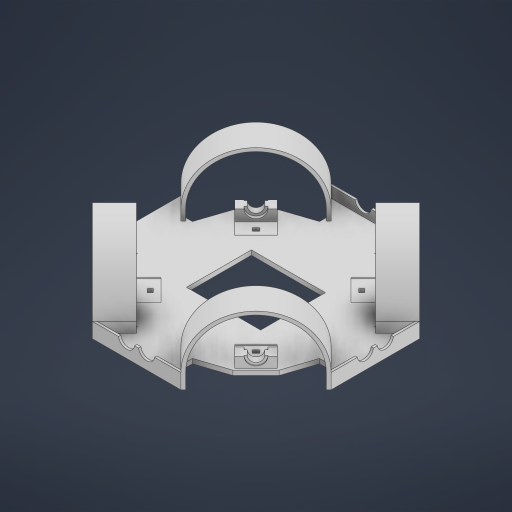
# Autodesk Inventor part: Robot Shell
Saved by Autodesk Inventor 2024 (Build 280153000, 153)
## iProperties
Created: 2025-11-14
Part Number: Robot Shell
Material: Generic
Document SubType Name: Modeling
Designer: Vincent Larson
Density: 1 g/cm^3
Appearance: Default
Author: Vincent Larson
Autodesk Inventor part; units mm, degrees
(part 1 of 2)
ref_plane "YZ Plane" through (0, 0, 0) normal (1, 0, 0) x (0, 1, 0)
ref_plane "XZ Plane" through (0, 0, 0) normal (0, 1, 0) x (-1, 0, 0)
ref_plane "XY Plane" through (0, 0, 0) normal (0, 0, 1) x (1, 0, 0)
sketch "Sketch1" plane through (0, 0, 0) normal (0, 1, 0) x (-1, 0, 0)
  line L0 (0, 0) -> (101.6, 0)
  line L1 (101.6, 0) -> (101.6, -203.2)
  line L2 (101.6, -203.2) -> (0, -203.2)
  line L3 (0, -203.2) -> (0, 0)
  line L4 (101.6, 0) -> (0, -203.2)
  line L5 (-50.8, -50.8) -> (152.4, -50.8)
  line L6 (152.4, -50.8) -> (152.4, -152.4)
  line L7 (152.4, -152.4) -> (-50.8, -152.4)
  line L8 (-50.8, -152.4) -> (-50.8, -50.8)
  line L9 (-50.8, -50.8) -> (152.4, -152.4) construction
  line L10 (152.4, -50.8) -> (-50.8, -152.4) construction
  line L11 (152.4, -152.4) -> (101.6, -203.2)
  line L12 (101.6, 0) -> (152.4, -50.8)
  line L13 (-50.8, -50.8) -> (0, 0)
  line L14 (0, -203.2) -> (-50.8, -152.4)
  point P0 (50.8, -101.6)
  point P1 (-50.8, -152.4)
  point P2 (152.4, -50.8)
  dimension "d0" = 101.6
  dimension "d1" = 203.2
  dimension "d2" = 203.2
  dimension "d3" = 101.6
  dimension "d6" = 360
  constraints: 30 end point, 4 parallel, 3 midpoint, 2 horizontal, 2 perpendicular, 17 other
  measures "d0" distance of L1.end L2.end
  measures "d1" distance of L0.end L1.end
  measures "d2" distance of L6.end L7.end
  measures "d3" distance of L5.end L6.end
extrude "Extrusion1" add sketch "Sketch1" along normal blind 5.08
sketch "Sketch2" plane through (0, 5.08, 0) normal (0, 1, 0) x (1, 0, 0)
  line L0 (0, 0) -> (50.8, 50.8) projected
  line L1 (0, 0) -> (50.8, 50.8)
  line L2 (50.8, 50.8) -> (25.4, 25.4)
  line L3 (25.4, 25.4) -> (-127, 177.8)
  line L4 (-101.6, 203.2) -> (-152.4, 152.4) projected
  line L5 (-50.8, 101.6) -> (-50.8, 0)
  line L6 (-101.6, 0) -> (0, 0) projected
  circle A0 centre (25.4, 25.4) radius 11.43
  line L7 (25.4, 25.4) -> (16.779, 34.021)
  line L8 (25.9388, 8.6967) -> (42.1033, 24.8612)
  line L9 (42.1033, 24.8612) -> (24.8612, 42.1033)
  line L10 (24.8612, 42.1033) -> (8.6967, 25.9388)
  line L11 (8.6967, 25.9388) -> (25.9388, 8.6967)
  line L12 (25.9388, 8.6967) -> (24.8612, 42.1033) construction
  line L13 (42.1033, 24.8612) -> (8.6967, 25.9388) construction
  line L14 (24.8612, 161.0967) -> (42.1033, 178.3388)
  line L15 (50.8, 152.4) -> (0, 203.2)
  line L16 (8.6967, 177.2612) -> (24.8612, 161.0967)
  line L17 (25.9388, 194.5033) -> (8.6967, 177.2612)
  line L18 (-110.2967, 177.2612) -> (-127.5388, 194.5033)
  line L19 (-101.6, 203.2) -> (-152.4, 152.4)
  line L20 (-126.4612, 161.0967) -> (-110.2967, 177.2612)
  line L21 (-143.7033, 178.3388) -> (-126.4612, 161.0967)
  line L22 (-126.4612, 42.1033) -> (-143.7033, 24.8612)
  line L23 (-152.4, 50.8) -> (-101.6, 0)
  line L24 (-110.2967, 25.9388) -> (-126.4612, 42.1033)
  line L25 (-127.5388, 8.6967) -> (-110.2967, 25.9388)
  line L26 (-112.2724, 23.9632) -> (-128.4368, 40.1276)
  line L27 (-128.4368, 40.1276) -> (-124.4855, 44.0789)
  line L28 (-124.4855, 44.0789) -> (-108.3211, 27.9145)
  line L29 (-108.3211, 27.9145) -> (-112.2724, 23.9632)
  line L30 (-112.2724, 23.9632) -> (-124.4855, 44.0789) construction
  line L31 (-128.4368, 40.1276) -> (-108.3211, 27.9145) construction
  line L32 (6.7211, 27.9145) -> (22.8855, 44.0789)
  line L33 (10.6724, 23.9632) -> (6.7211, 27.9145)
  line L34 (22.8855, 44.0789) -> (26.8368, 40.1276)
  line L35 (22.8855, 159.1211) -> (6.7211, 175.2855)
  line L36 (26.8368, 163.0724) -> (22.8855, 159.1211)
  line L37 (6.7211, 175.2855) -> (10.6724, 179.2368)
  line L38 (-108.3211, 175.2855) -> (-124.4855, 159.1211)
  line L39 (-112.2724, 179.2368) -> (-108.3211, 175.2855)
  line L40 (-124.4855, 159.1211) -> (-128.4368, 163.0724)
  point P0 (25.4, 177.8)
  point P1 (-127, 177.8)
  point P2 (-127, 25.4)
  point P3 (17.3178, 17.3178)
  point P4 (33.4822, 33.4822)
  point P5 (33.4822, 169.7178)
  point P6 (17.3178, 185.8822)
  point P7 (-135.0822, 169.7178)
  point P8 (-118.9178, 185.8822)
  point P9 (-135.0822, 33.4822)
  point P10 (-118.9178, 17.3178)
  point P11 (-118.379, 34.021)
  dimension "d10" = 22.86
  dimension "d11" = 12.192
  dimension "d14" = 360
  dimension "d38" = 5.588
  dimension "d41" = 360
  constraints: 76 end point, 9 midpoint, 6 equal length, 2 perpendicular, 1 centre point, 1 coincident, 1 point on line, 74 other
  measures "d10" diameter of A0
  measures "d11" distance of L7.start L7.end
  measures "d38" distance of L26.end L27.end
extrude "Extrusion2" add sketch "Sketch2" along normal blind 25.4 contours A0 L3 L0 | L11 L10 L3 A0 | L3 A0 L0 | L3 L10 L9 A0 | L10 L33 L32 L3 | L3 L32 L34 L10 | L38 L40 L20 L3 | L3 L20 L39 L38 | L20 L21 L4 L3 | L3 L4 L18 L20 | L16 L17 L15 L14 | L36 L35 L37 L16 | L24 L25 L26 L22 | L27 L28 L29 L24 | L26 L25 L23 L22
sketch "Sketch3" plane through (50.8, 0, -50.8) normal (0.7071068, 0, 0.7071068) x (0.7071068, 0, -0.7071068)
  line L0 (-24.491, 5.08) -> (-47.351, 5.08) projected
  line L1 (-35.921, 5.08) -> (-35.921, 7.62)
  line L2 (-35.921, 7.62) -> (-35.921, 25.4)
  circle A0 centre (-35.921, 16.51) radius 9.271
  line L3 (-47.351, 5.08) -> (-47.351, 30.48) projected
  line L4 (-47.351, 16.51) -> (-16.699, 16.51)
  line L5 (-16.699, 16.51) -> (-16.699, 33.825)
  line L6 (-16.699, 33.825) -> (-47.351, 33.825)
  line L7 (-47.351, 33.825) -> (-47.351, 16.51)
  point P0 (-71.842, 0)
  point P1 (-45.192, 16.51)
  point P2 (-26.65, 16.51)
  point P3 (-47.351, 30.48)
  dimension "d18" = 2.54
  dimension "d19" = 17.78
  dimension "d20" = 18.542
  constraints: 12 end point, 2 midpoint, 2 parallel, 2 point on line, 1 centre point, 1 horizontal, 1 perpendicular, 1 vertical
  measures "d18" distance of L1.start L1.end
  measures "d19" distance of L1.end L2.end
  measures "d20" diameter of A0
extrude "Extrusion3" cut sketch "Sketch3" against normal through all contours A0 L4 L2 L1 | L1 L2 L4 A0 | L3 L7 L6 L5 L4 A0 | A0 L4
sketch "Sketch4" plane through (0, 0, -203.2) normal (0.7071068, 0, -0.7071068) x (-0.7071068, 0, -0.7071068)
  line L0 (-24.491, 30.48) -> (-47.351, 30.48) projected
  line L1 (-47.351, 5.08) -> (-24.491, 5.08) projected
  line L2 (-47.351, 30.48) -> (-24.491, 30.48)
  line L3 (-24.491, 30.48) -> (-24.491, 5.08)
  line L4 (-24.491, 5.08) -> (-47.351, 5.08)
  line L5 (-47.351, 5.08) -> (-47.351, 30.48)
  circle A0 centre (-35.921, 16.51) radius 9.271
  line L6 (-75.7535, 47.6212) -> (-19.9312, 47.6212)
  line L7 (-19.9312, 47.6212) -> (-19.9312, 16.51)
  line L8 (-19.9312, 16.51) -> (-75.7535, 16.51)
  line L9 (-75.7535, 16.51) -> (-75.7535, 47.6212)
  point P0 (-143.6841, 0)
  point P1 (-45.192, 16.51)
  point P2 (-26.65, 16.51)
  point P3 (-24.491, 16.51)
  point P4 (-24.491, 30.48)
  point P5 (-47.351, 16.51)
  constraints: 16 end point, 4 parallel, 2 horizontal, 2 perpendicular, 1 centre point
extrude "Extrusion4" cut sketch "Sketch4" against normal through all contours L3 L8 A0 L5 L0 | L8 A0 | A0 L8
sketch "Sketch5" plane through (0, 5.08, 0) normal (0, 1, 0) x (1, 0, 0)
  line L0 (-152.4, 152.4) -> (-152.4, 50.8) projected
  line L1 (-152.4, 101.6) -> (50.8, 101.6)
  line L2 (50.8, 50.8) -> (50.8, 152.4) projected
  line L3 (-50.8, 101.6) -> (-127, 25.4)
  line L4 (-152.4, 50.8) -> (-101.6, 0) projected
  line L5 (-112.4905, 7.2984) -> (-145.1016, 39.9095)
  line L6 (-145.1016, 39.9095) -> (-141.5095, 43.5016)
  line L7 (-141.5095, 43.5016) -> (-108.8984, 10.8905)
  line L8 (-108.8984, 10.8905) -> (-112.4905, 7.2984)
  line L9 (-112.4905, 7.2984) -> (-141.5095, 43.5016) construction
  line L10 (-145.1016, 39.9095) -> (-108.8984, 10.8905) construction
  line L11 (43.5016, 39.9095) -> (10.8905, 7.2984)
  line L12 (10.8905, 7.2984) -> (7.2984, 10.8905)
  line L13 (7.2984, 10.8905) -> (39.9095, 43.5016)
  line L14 (39.9095, 43.5016) -> (43.5016, 39.9095)
  line L15 (43.5016, 39.9095) -> (7.2984, 10.8905) construction
  line L16 (10.8905, 7.2984) -> (39.9095, 43.5016) construction
  line L17 (10.8905, 195.9016) -> (43.5016, 163.2905)
  line L18 (43.5016, 163.2905) -> (39.9095, 159.6984)
  line L19 (39.9095, 159.6984) -> (7.2984, 192.3095)
  line L20 (7.2984, 192.3095) -> (10.8905, 195.9016)
  line L21 (10.8905, 195.9016) -> (39.9095, 159.6984) construction
  line L22 (43.5016, 163.2905) -> (7.2984, 192.3095) construction
  line L23 (-145.1016, 163.2905) -> (-112.4905, 195.9016)
  line L24 (-112.4905, 195.9016) -> (-108.8984, 192.3095)
  line L25 (-108.8984, 192.3095) -> (-141.5095, 159.6984)
  line L26 (-141.5095, 159.6984) -> (-145.1016, 163.2905)
  line L27 (-145.1016, 163.2905) -> (-108.8984, 192.3095) construction
  line L28 (-112.4905, 195.9016) -> (-141.5095, 159.6984) construction
  point P0 (0, 0)
  point P1 (0, 0)
  point P2 (25.4, 25.4)
  point P3 (50.8, 152.4)
  point P4 (25.4, 177.8)
  point P5 (-101.6, 203.2)
  point P6 (-127, 177.8)
  dimension "d25" = 5.08
  dimension "d28" = 360
  constraints: 52 end point, 12 midpoint, 2 coincident, 2 parallel, 1 perpendicular, 51 other
  measures "d25" distance of L5.end L6.end
extrude "Extrusion5" cut sketch "Sketch5" along normal blind 25.4 contours L6 L7 L3 L4 | L4 L8 L5 L6 | L7 L8 L4 L3 | L11 L12 L13 L14 | L17 L18 L19 L20 | L23 L24 L25 L26
sketch "Sketch6" plane through (0, 5.08, 0) normal (0, 1, 0) x (1, 0, 0)
  line L0 (0, 0) -> (50.8, 50.8) projected
  line L1 (25.4, 25.4) -> (50.8, 50.8)
  line L2 (50.8, 50.8) -> (38.1, 38.1)
  line L3 (50.8, 50.8) -> (50.8, 152.4) projected
  line L4 (50.8, 50.8) -> (50.8, 152.4)
  line L5 (50.8, 152.4) -> (50.8, 101.6)
  line L6 (50.8, 101.6) -> (50.8, 50.8)
  line L7 (50.8, 76.2) -> (38.1, 38.1)
  line L8 (25.4, 25.4) -> (0, 0)
  line L9 (-101.6, 0) -> (0, 0) projected
  line L10 (0, 0) -> (-101.6, 0)
  line L11 (-101.6, 0) -> (-50.8, 0)
  line L12 (-50.8, 0) -> (0, 0)
  line L13 (-25.4, 0) -> (12.7, 12.7)
  line L14 (-50.8, 0) -> (-50.8, 101.6)
  line L15 (-50.8, 101.6) -> (50.8, 101.6)
  line L16 (50.8, 127) -> (38.1, 165.1)
  line L17 (-25.4, 203.2) -> (12.7, 190.5)
  line L18 (0, 203.2) -> (-101.6, 203.2)
  line L19 (25.4, 177.8) -> (0, 203.2)
  line L20 (25.4, 177.8) -> (50.8, 152.4)
  line L21 (50.8, 152.4) -> (50.8, 50.8)
  line L22 (-76.2, 203.2) -> (-114.3, 190.5)
  line L23 (-152.4, 127) -> (-139.7, 165.1)
  line L24 (-152.4, 152.4) -> (-152.4, 50.8)
  line L25 (-127, 177.8) -> (-152.4, 152.4)
  line L26 (-127, 177.8) -> (-101.6, 203.2)
  line L27 (-101.6, 203.2) -> (0, 203.2)
  line L28 (-152.4, 76.2) -> (-139.7, 38.1)
  line L29 (-76.2, 0) -> (-114.3, 12.7)
  line L30 (-101.6, 0) -> (0, 0)
  line L31 (-127, 25.4) -> (-101.6, 0)
  line L32 (-127, 25.4) -> (-152.4, 50.8)
  line L33 (-152.4, 50.8) -> (-152.4, 152.4)
  point P0 (-50.8, 203.2)
  point P1 (50.8, 101.6)
  point P2 (-152.4, 101.6)
  point P3 (-50.8, 203.2)
  point P4 (-50.8, 0)
  point P5 (-152.4, 101.6)
  dimension "d34" = 360
  constraints: 62 end point, 7 midpoint, 6 collinear, 1 perpendicular, 1 vertical, 69 other
extrude "Extrusion6" cut sketch "Sketch6" against normal blind 25.4 contours L9 L13 L0 | L7 L3 L0 | L9 L31 L29 | L16 L20 L3 | L32 L24 L28 | L24 L25 L23 | L17 L18 L19 | L22 L26 L18
ref_plane "Work Plane1" through (14.7315, 5.08, -19.9041) normal (0.7071068, 0, 0.7071068) x (0.7071068, 0, -0.7071068)
sketch "Sketch7" plane through (14.7315, 5.08, -19.9041) normal (0.7071068, 0, 0.7071068) x (0.7071068, 0, -0.7071068)
  arc A0 (2.159, 11.43) -> (20.701, 11.43) centre (11.43, 11.43) ccw projected
  circle A1 centre (11.43, 11.43) radius 9.271
  arc A2 (4.699, 11.43) -> (18.161, 11.43) centre (11.43, 11.43) ccw
  line L0 (0, 0) -> (0, 11.43) projected
  line L1 (0, 11.43) -> (22.7953, 11.43)
  point P0 (-24.491, -5.08)
  point P1 (4.699, 11.43)
  point P2 (2.159, 11.43)
  point P3 (20.701, 11.43)
  point P4 (18.161, 11.43)
  dimension "d44" = 2.54
  constraints: 2 centre point, 2 end point, 2 point on circle, 1 coincident, 1 perpendicular
  measures "d44" radial gap between concentric circles of A0 A2
extrude "Extrusion7" add sketch "Sketch7" against normal blind 7.62 contours L1 A2 A0
sketch "Sketch8" plane through (0, 5.08, 0) normal (0, 1, 0) x (1, 0, 0)
  line L0 (-124.4855, 44.0789) -> (-122.9589, 42.5523) projected
  line L1 (-117.1217, 19.1138) -> (-133.2862, 35.2783) projected
  line L2 (-124.4855, 44.0789) -> (-133.2862, 35.2783)
  line L3 (-133.2862, 35.2783) -> (-136.8783, 38.8704)
  line L4 (-136.8783, 38.8704) -> (-128.0776, 47.671)
  line L5 (-128.0776, 47.671) -> (-124.4855, 44.0789)
  line L6 (-108.3211, 27.9145) -> (-117.1217, 19.1138) projected
  line L7 (-108.3211, 27.9145) -> (-117.1217, 19.1138)
  line L8 (-117.1217, 19.1138) -> (-113.5296, 15.5217)
  line L9 (-113.5296, 15.5217) -> (-104.729, 24.3224)
  line L10 (-104.729, 24.3224) -> (-108.3211, 27.9145)
  line L11 (-122.9589, 42.5523) -> (-131.7595, 33.7516) projected
  line L12 (-131.7595, 33.7516) -> (-130.9693, 34.5419)
  line L13 (-130.9693, 34.5419) -> (-117.8581, 21.4307)
  line L14 (-109.8477, 29.4411) -> (-118.6484, 20.6405) projected
  line L15 (-117.8581, 21.4307) -> (-112.4699, 26.8189)
  line L16 (-112.4699, 26.8189) -> (-125.5811, 39.9301)
  line L17 (-125.5811, 39.9301) -> (-130.9693, 34.5419)
  line L18 (-122.9589, 42.5523) -> (-109.8477, 29.4411) projected
  line L19 (-116.4033, 35.9967) -> (14.8033, 167.2033)
  line L20 (21.3589, 160.6477) -> (8.2477, 173.7589) projected
  line L21 (-50.8, 101.6) -> (-50.8, 0)
  line L22 (-76.2, 0) -> (-25.4, 0) projected
  line L23 (23.9811, 39.9301) -> (10.8699, 26.8189)
  line L24 (16.2581, 21.4307) -> (29.3693, 34.5419)
  line L25 (29.3693, 34.5419) -> (23.9811, 39.9301)
  line L26 (31.6862, 35.2783) -> (35.2783, 38.8704)
  line L27 (22.8855, 44.0789) -> (31.6862, 35.2783)
  line L28 (10.8699, 26.8189) -> (16.2581, 21.4307)
  line L29 (3.129, 24.3224) -> (6.7211, 27.9145)
  line L30 (6.7211, 27.9145) -> (15.5217, 19.1138)
  line L31 (15.5217, 19.1138) -> (11.9296, 15.5217)
  line L32 (11.9296, 15.5217) -> (3.129, 24.3224)
  line L33 (17.0484, 20.6405) -> (16.2581, 21.4307)
  line L34 (26.4776, 47.671) -> (22.8855, 44.0789)
  line L35 (35.2783, 38.8704) -> (26.4776, 47.671)
  line L36 (10.8699, 176.3811) -> (23.9811, 163.2699)
  line L37 (29.3693, 168.6581) -> (16.2581, 181.7693)
  line L38 (16.2581, 181.7693) -> (10.8699, 176.3811)
  line L39 (15.5217, 184.0862) -> (11.9296, 187.6783)
  line L40 (6.7211, 175.2855) -> (15.5217, 184.0862)
  line L41 (23.9811, 163.2699) -> (29.3693, 168.6581)
  line L42 (26.4776, 155.529) -> (22.8855, 159.1211)
  line L43 (22.8855, 159.1211) -> (31.6862, 167.9217)
  line L44 (31.6862, 167.9217) -> (35.2783, 164.3296)
  line L45 (35.2783, 164.3296) -> (26.4776, 155.529)
  line L46 (30.1595, 169.4484) -> (29.3693, 168.6581)
  line L47 (3.129, 178.8776) -> (6.7211, 175.2855)
  line L48 (11.9296, 187.6783) -> (3.129, 178.8776)
  line L49 (-125.5811, 163.2699) -> (-112.4699, 176.3811)
  line L50 (-117.8581, 181.7693) -> (-130.9693, 168.6581)
  line L51 (-130.9693, 168.6581) -> (-125.5811, 163.2699)
  line L52 (-133.2862, 167.9217) -> (-136.8783, 164.3296)
  line L53 (-124.4855, 159.1211) -> (-133.2862, 167.9217)
  line L54 (-112.4699, 176.3811) -> (-117.8581, 181.7693)
  line L55 (-104.729, 178.8776) -> (-108.3211, 175.2855)
  line L56 (-108.3211, 175.2855) -> (-117.1217, 184.0862)
  line L57 (-117.1217, 184.0862) -> (-113.5296, 187.6783)
  line L58 (-113.5296, 187.6783) -> (-104.729, 178.8776)
  line L59 (-118.6484, 182.5595) -> (-117.8581, 181.7693)
  line L60 (-128.0776, 155.529) -> (-124.4855, 159.1211)
  line L61 (-136.8783, 164.3296) -> (-128.0776, 155.529)
  point P0 (0, 0)
  point P1 (14.8033, 35.9967)
  point P2 (14.8033, 167.2033)
  point P3 (-116.4033, 167.2033)
  dimension "d47" = 5.08
  dimension "d48" = 5.08
  dimension "d49" = 1.1176
  dimension "d50" = 7.62
  dimension "d53" = 360
  constraints: 108 end point, 7 point on line, 5 perpendicular, 4 midpoint, 4 parallel, 2 collinear, 109 other
  measures "d47" distance of L1.end L3.end
  measures "d48" distance of L8.end L1.start
  measures "d49" distance of L11.end L12.end
  measures "d50" distance of L13.end L15.end
extrude "Extrusion8" add sketch "Sketch8" along normal up to surface (11.43 mm away) contours L0 L11 L1 L2 | L2 L3 L4 L5 | L16 L14 L13 L11 | L10 L9 L8 L6 | L25 L24 L28 L23 | L27 L34 L35 L26 | L29 L30 L31 L32 | L38 L37 L41 L36 | L40 L47 L48 L39 | L42 L43 L44 L45 | L51 L50 L54 L49 | L53 L60 L61 L52 | L55 L56 L57 L58
sketch "Sketch9" plane through (14.7315, 5.08, -19.9041) normal (0.7071068, 0, 0.7071068) x (0.7071068, 0, -0.7071068)
  line L0 (2.159, 11.43) -> (20.701, 11.43) projected
  circle A0 centre (11.43, 11.43) radius 9.271
  circle A1 centre (11.43, 11.43) radius 6.731
  point P0 (-24.491, -5.08)
  dimension "d57" = 2.54
  constraints: 2 centre point, 1 midpoint
  measures "d57" radial gap between concentric circles of A0 A1
extrude "Extrusion9" cut sketch "Sketch9" against normal through all contours A1 L0 | L0 A1
sketch "Sketch10" plane through (22.8137, 16.51, -175.2137) normal (0.7071068, 0, -0.7071068) x (-0.7071068, 0, -0.7071068)
  line L0 (16.51, 0) -> (-16.51, 0) projected
  circle A0 centre (0, 0) radius 6.731
  point P0 (-107.7631, -16.51)
  point P1 (-6.731, 0)
  point P2 (6.731, 0)
  dimension "d60" = 13.462
  constraints: 1 centre point, 1 midpoint
  measures "d60" diameter of A0
extrude "Extrusion10" cut sketch "Sketch10" against normal through all contours A0 L0 picked at (-0.7304, -2.6348)
sketch "Sketch11" plane through (0, 5.08, 0) normal (0, 1, 0) x (1, 0, 0)
  line L0 (-122.9589, 42.5523) -> (-128.0776, 47.671) projected
  line L1 (-104.729, 24.3224) -> (-113.5296, 15.5217) projected
  line L2 (-128.0776, 47.671) -> (-104.729, 24.3224)
  line L3 (-104.729, 24.3224) -> (-91.2586, 37.7928)
  line L4 (-91.2586, 37.7928) -> (-114.6072, 61.1414)
  line L5 (-114.6072, 61.1414) -> (-128.0776, 47.671)
  line L6 (-102.9329, 49.4671) -> (14.8033, 167.2033)
  line L7 (26.4776, 155.529) -> (3.129, 178.8776) projected
  line L8 (-76.2, 0) -> (-25.4, 0) projected
  line L9 (-50.8, 0) -> (-50.8, 203.2)
  line L10 (-25.4, 203.2) -> (-76.2, 203.2) projected
  circle A0 centre (-50.8, 101.6) radius 24.6692
  line L11 (13.0072, 61.1414) -> (-10.3414, 37.7928)
  line L12 (26.4776, 47.671) -> (13.0072, 61.1414)
  line L13 (3.129, 24.3224) -> (26.4776, 47.671)
  line L14 (-10.3414, 37.7928) -> (3.129, 24.3224)
  line L15 (-10.3414, 165.4072) -> (13.0072, 142.0586)
  line L16 (3.129, 178.8776) -> (-10.3414, 165.4072)
  line L17 (26.4776, 155.529) -> (3.129, 178.8776)
  line L18 (13.0072, 142.0586) -> (26.4776, 155.529)
  line L19 (-114.6072, 142.0586) -> (-91.2586, 165.4072)
  line L20 (-128.0776, 155.529) -> (-114.6072, 142.0586)
  line L21 (-104.729, 178.8776) -> (-128.0776, 155.529)
  line L22 (-91.2586, 165.4072) -> (-104.729, 178.8776)
  point P0 (0, 0)
  point P1 (1.3329, 49.4671)
  point P2 (1.3329, 153.7329)
  point P3 (-102.9329, 153.7329)
  dimension "d63" = 19.05
  dimension "d66" = 360
  constraints: 36 end point, 5 midpoint, 2 parallel, 2 perpendicular, 1 centre point, 37 other
  measures "d63" distance of L3.end L1.start
extrude "Extrusion11" cut sketch "Sketch11" against normal blind 0.508 contours L0 L5 L4 L3 L2 | L15 L16 L7 L6 | L6 L7 L18 L15 | L12 L13 L14 L11 | L20 L21 L22 L19
sketch "Sketch12" plane through (0, 4.572, 0) normal (0, 1, 0) x (1, 0, 0)
  line L0 (8.2477, 29.4411) -> (21.3589, 42.5523) projected
  line L1 (14.8033, 35.9967) -> (8.8763, 41.9237)
  line L2 (14.8033, 35.9967) -> (23.1853, 35.9967) construction
  line L3 (-10.3414, 37.7928) -> (13.0072, 61.1414) projected
  line L4 (1.3329, 49.4671) -> (5.6434, 45.1566)
  line L5 (1.3329, 49.4671) -> (7.4289, 49.4671) construction
  line L6 (8.8763, 41.9237) -> (5.6434, 45.1566)
  line L7 (6.9007, 39.948) -> (3.6678, 43.1809)
  line L8 (3.6678, 43.1809) -> (7.6191, 47.1322)
  line L9 (7.6191, 47.1322) -> (10.852, 43.8993)
  line L10 (10.852, 43.8993) -> (6.9007, 39.948)
  line L11 (6.9007, 39.948) -> (7.6191, 47.1322) construction
  line L12 (3.6678, 43.1809) -> (10.852, 43.8993) construction
  line L13 (-76.2, 0) -> (-25.4, 0) projected
  line L14 (-50.8, 0) -> (-50.8, 203.2)
  line L15 (-25.4, 203.2) -> (-76.2, 203.2) projected
  line L16 (50.8, 76.2) -> (50.8, 127) projected
  line L17 (50.8, 101.6) -> (-50.8, 101.6)
  circle A0 centre (-50.8, 101.6) radius 124.16
  line L18 (14.8033, 167.2033) -> (8.8763, 161.2763)
  line L19 (6.9007, 163.252) -> (10.852, 159.3007)
  line L20 (3.6678, 160.0191) -> (6.9007, 163.252)
  line L21 (8.8763, 161.2763) -> (5.6434, 158.0434)
  line L22 (7.6191, 156.0678) -> (6.9007, 163.252) construction
  line L23 (1.3329, 153.7329) -> (5.6434, 158.0434)
  line L24 (1.3329, 153.7329) -> (1.3329, 159.8289) construction
  line L25 (10.852, 159.3007) -> (7.6191, 156.0678)
  line L26 (7.6191, 156.0678) -> (3.6678, 160.0191)
  line L27 (10.852, 159.3007) -> (3.6678, 160.0191) construction
  line L28 (-116.4033, 167.2033) -> (-110.4763, 161.2763)
  line L29 (-112.452, 159.3007) -> (-108.5007, 163.252)
  line L30 (-109.2191, 156.0678) -> (-112.452, 159.3007)
  line L31 (-110.4763, 161.2763) -> (-107.2434, 158.0434)
  line L32 (-105.2678, 160.0191) -> (-112.452, 159.3007) construction
  line L33 (-102.9329, 153.7329) -> (-107.2434, 158.0434)
  line L34 (-102.9329, 153.7329) -> (-109.0289, 153.7329) construction
  line L35 (-108.5007, 163.252) -> (-105.2678, 160.0191)
  line L36 (-105.2678, 160.0191) -> (-109.2191, 156.0678)
  line L37 (-108.5007, 163.252) -> (-109.2191, 156.0678) construction
  line L38 (-116.4033, 35.9967) -> (-110.4763, 41.9237)
  line L39 (-108.5007, 39.948) -> (-112.452, 43.8993)
  line L40 (-105.2678, 43.1809) -> (-108.5007, 39.948)
  line L41 (-110.4763, 41.9237) -> (-107.2434, 45.1566)
  line L42 (-109.2191, 47.1322) -> (-108.5007, 39.948) construction
  line L43 (-102.9329, 49.4671) -> (-107.2434, 45.1566)
  line L44 (-102.9329, 49.4671) -> (-102.9329, 43.3711) construction
  line L45 (-112.452, 43.8993) -> (-109.2191, 47.1322)
  line L46 (-109.2191, 47.1322) -> (-105.2678, 43.1809)
  line L47 (-112.452, 43.8993) -> (-105.2678, 43.1809) construction
  point P0 (0, 0)
  point P1 (7.2599, 43.5401)
  point P2 (7.2599, 159.6599)
  point P3 (-108.8599, 159.6599)
  point P4 (-108.8599, 43.5401)
  dimension "d70" = 8.382
  dimension "d71" = 135
  dimension "d72" = 6.096
  dimension "d73" = 45
  dimension "d74" = 5.588
  dimension "d79" = 360
  constraints: 86 end point, 15 midpoint, 3 parallel, 3 perpendicular, 2 equal length, 2 horizontal, 1 centre point, 1 coincident, 81 other
  measures "d70" distance of L1.start L1.end
  measures "d71" angle of L2 L1
  measures "d72" distance of L4.start L4.end
  measures "d73" angle of L4 L5
  measures "d74" distance of L7.end L8.end
extrude "Extrusion12" cut sketch "Sketch12" against normal blind 14.7955 contours L10 L7 L8 L6 | L6 L8 L9 L10 | L19 L21 L26 L20 | L19 L25 L26 L21 | L29 L31 L36 L30 | L29 L35 L36 L31 | L39 L41 L46 L40 | L39 L45 L46 L41
sketch "Sketch13" plane through (0, 5.08, 0) normal (0, 1, 0) x (1, 0, 0)
  line L0 (-10.3414, 37.7928) -> (13.0072, 61.1414) projected
  line L1 (1.3329, 49.4671) -> (-102.9329, 153.7329)
  line L2 (-91.2586, 165.4072) -> (-114.6072, 142.0586) projected
  line L3 (13.0072, 142.0586) -> (-10.3414, 165.4072) projected
  line L4 (1.3329, 153.7329) -> (-102.9329, 49.4671)
  line L5 (-91.44, 66.04) -> (-10.16, 66.04)
  line L6 (-10.16, 66.04) -> (-10.16, 137.16)
  line L7 (-10.16, 137.16) -> (-91.44, 137.16)
  line L8 (-91.44, 137.16) -> (-91.44, 66.04)
  line L9 (-91.44, 66.04) -> (-10.16, 137.16) construction
  line L10 (-10.16, 66.04) -> (-91.44, 137.16) construction
  point P0 (0, 0)
  point P1 (-50.8, 101.6)
  dimension "d81" = 81.28
  dimension "d82" = 71.12
  constraints: 16 end point, 6 midpoint, 2 parallel, 2 perpendicular, 1 horizontal
  measures "d81" distance of L5.start L5.end
  measures "d82" distance of L6.end L5.end
extrude "Extrusion13" cut sketch "Sketch13" against normal blind 25.4
sketch "Sketch14" plane through (0, 5.08, 0) normal (0, 1, 0) x (1, 0, 0)
  line L0 (-72.39, 207.01) -> (-29.21, 207.01)
  line L1 (-29.21, 207.01) -> (-29.21, 199.39)
  line L2 (-29.21, 199.39) -> (-72.39, 199.39)
  line L3 (-72.39, 199.39) -> (-72.39, 207.01)
  line L4 (-25.4, 203.2) -> (-76.2, 203.2) projected
  line L5 (-72.39, 207.01) -> (-29.21, 199.39) construction
  line L6 (-29.21, 207.01) -> (-72.39, 199.39) construction
  line L7 (-10.16, 137.16) -> (-10.16, 66.04) projected
  line L8 (-10.16, 66.04) -> (-91.44, 66.04) projected
  line L9 (-10.16, 137.16) -> (-91.44, 66.04)
  line L10 (-91.44, 66.04) -> (-91.44, 137.16)
  line L11 (-91.44, 137.16) -> (-10.16, 66.04)
  circle A0 centre (-50.8, 101.6) radius 22.6578
  line L12 (-156.21, 80.01) -> (-156.21, 123.19)
  line L13 (-156.21, 123.19) -> (-148.59, 123.19)
  line L14 (-148.59, 123.19) -> (-148.59, 80.01)
  line L15 (-148.59, 80.01) -> (-156.21, 80.01)
  line L16 (-156.21, 80.01) -> (-148.59, 123.19) construction
  line L17 (-156.21, 123.19) -> (-148.59, 80.01) construction
  line L18 (-29.21, -3.81) -> (-72.39, -3.81)
  line L19 (-72.39, -3.81) -> (-72.39, 3.81)
  line L20 (-72.39, 3.81) -> (-29.21, 3.81)
  line L21 (-29.21, 3.81) -> (-29.21, -3.81)
  line L22 (-29.21, -3.81) -> (-72.39, 3.81) construction
  line L23 (-72.39, -3.81) -> (-29.21, 3.81) construction
  line L24 (54.61, 123.19) -> (54.61, 80.01)
  line L25 (54.61, 80.01) -> (46.99, 80.01)
  line L26 (46.99, 80.01) -> (46.99, 123.19)
  line L27 (46.99, 123.19) -> (54.61, 123.19)
  line L28 (54.61, 123.19) -> (46.99, 80.01) construction
  line L29 (54.61, 80.01) -> (46.99, 123.19) construction
  line L30 (-152.4, 0) -> (50.8, 0)
  line L31 (50.8, 0) -> (50.8, 203.2)
  line L32 (50.8, 203.2) -> (-152.4, 203.2)
  line L33 (-152.4, 203.2) -> (-152.4, 0)
  line L34 (-152.4, 0) -> (50.8, 203.2) construction
  line L35 (50.8, 0) -> (-152.4, 203.2) construction
  line L36 (-148.59, 80.01) -> (-156.21, 80.01)
  line L37 (-156.21, 80.01) -> (-156.21, 123.19)
  line L38 (-156.21, 123.19) -> (-148.59, 123.19)
  line L39 (-148.59, 123.19) -> (-148.59, 80.01)
  line L40 (-148.59, 80.01) -> (-156.21, 123.19) construction
  line L41 (-156.21, 80.01) -> (-148.59, 123.19) construction
  line L42 (-156.21, 76.2) -> (-148.59, 76.2)
  line L43 (-148.59, 76.2) -> (-148.59, 127)
  line L44 (-148.59, 127) -> (-156.21, 127)
  line L45 (-156.21, 127) -> (-156.21, 76.2)
  line L46 (-156.21, 76.2) -> (-148.59, 127) construction
  line L47 (-148.59, 76.2) -> (-156.21, 127) construction
  line L48 (-25.4, -3.81) -> (-76.2, -3.81)
  line L49 (-76.2, -3.81) -> (-76.2, 3.81)
  line L50 (-76.2, 3.81) -> (-25.4, 3.81)
  line L51 (-25.4, 3.81) -> (-25.4, -3.81)
  line L52 (-25.4, -3.81) -> (-76.2, 3.81) construction
  line L53 (-76.2, -3.81) -> (-25.4, 3.81) construction
  line L54 (-25.4, 199.39) -> (-76.2, 199.39)
  line L55 (-76.2, 199.39) -> (-76.2, 207.01)
  line L56 (-76.2, 207.01) -> (-25.4, 207.01)
  line L57 (-25.4, 207.01) -> (-25.4, 199.39)
  line L58 (-25.4, 199.39) -> (-76.2, 207.01) construction
  line L59 (-76.2, 199.39) -> (-25.4, 207.01) construction
  point P0 (0, 0)
  point P1 (-50.8, 203.2)
  point P2 (-152.4, 101.6)
  point P3 (-50.8, 0)
  point P4 (50.8, 101.6)
  point P5 (-29.21, 203.2)
  point P6 (-72.39, 203.2)
  point P7 (50.8, 80.01)
  point P8 (50.8, 123.19)
  point P9 (-72.39, 0)
  point P10 (-29.21, 0)
  point P11 (-152.4, 123.19)
  point P12 (-152.4, 80.01)
  point P13 (-152.4, 76.2)
  point P14 (-152.4, 127)
  point P15 (-25.4, 0)
  point P16 (-76.2, 0)
  dimension "d85" = 43.18
  dimension "d86" = 7.62
  dimension "d89" = 360
  constraints: 114 end point, 14 midpoint, 12 parallel, 7 perpendicular, 6 horizontal, 2 point on line, 1 centre point, 45 other
  measures "d85" distance of L1.end L2.end
  measures "d86" distance of L0.end L1.end
extrude "Extrusion14" add sketch "Sketch14" along normal blind 25.4 contours L4 L1 L2 L3 | L3 L54 L55 L4 | L4 L57 L54 L1 | L44 L43 L13 L33 | L31 L25 L26 L27 | L13 L14 L15 L33 | L15 L43 L42 L33 | L30 L21 L50 L51 | L30 L19 L20 L21 | L49 L50 L19 L30
sketch "Sketch15" plane through (0, 5.08, 0) normal (0, 1, 0) x (1, 0, 0)
  line L0 (46.99, 80.01) -> (46.99, 123.19) projected
  line L1 (50.8, 80.01) -> (46.99, 80.01) projected
  line L2 (46.99, 123.19) -> (50.8, 123.19)
  line L3 (50.8, 123.19) -> (50.8, 80.01)
  line L4 (50.8, 80.01) -> (46.99, 80.01)
  line L5 (46.99, 80.01) -> (46.99, 123.19)
  line L6 (50.8, 76.2) -> (50.8, 127) projected
  line L7 (46.99, 76.2) -> (50.8, 76.2)
  line L8 (50.8, 76.2) -> (50.8, 127)
  line L9 (50.8, 127) -> (46.99, 127)
  line L10 (46.99, 127) -> (46.99, 76.2)
  line L11 (46.99, 76.2) -> (50.8, 127) construction
  line L12 (50.8, 76.2) -> (46.99, 127) construction
  point P0 (0, 0)
  point P1 (48.895, 101.6)
  constraints: 20 end point, 4 parallel, 2 horizontal, 2 midpoint, 2 perpendicular
extrude "Extrusion15" add sketch "Sketch15" along normal blind 25.4
sketch "Sketch17" plane through (0, 5.08, 0) normal (0, 1, 0) x (1, 0, 0)
  line L0 (-121.3031, 70.7582) -> (-170.5024, 70.7582)
  line L1 (-170.5024, 70.7582) -> (-170.5024, 134.465)
  line L2 (-170.5024, 134.465) -> (-121.3031, 134.465)
  line L3 (-121.3031, 134.465) -> (-121.3031, 70.7582)
  line L4 (-121.3031, 70.7582) -> (-170.5024, 134.465) construction
  line L5 (-170.5024, 70.7582) -> (-121.3031, 134.465) construction
  point P0 (0, 0)
  point P1 (-145.9028, 102.6116)
  constraints: 12 end point, 2 midpoint, 2 parallel, 1 horizontal, 1 perpendicular
extrude "Extrusion16" cut sketch "Sketch17" along normal blind 25.4
sketch "Sketch18" plane through (-76.2, 0, 0) normal (0, 0, 1) x (1, 0, 0)
  line L0 (-15.24, 5.08) -> (66.04, 5.08) projected
  line L1 (25.4, 5.08) -> (25.4, 30.48)
  line L2 (50.8, 30.48) -> (0, 30.48) projected
  circle A0 centre (25.4, 17.78) radius 8.4963
  line L3 (25.4, 17.78) -> (14.1478, 17.78)
  circle A1 centre (14.1478, 17.78) radius 8.89
  circle A2 centre (36.6522, 17.78) radius 8.89
  point P0 (76.2, 0)
  dimension "d97" = 16.9926
  dimension "d98" = 11.2522
  dimension "d99" = 17.78
  constraints: 4 end point, 3 centre point, 3 midpoint, 1 coincident, 1 horizontal, 1 symmetric about line, 1 other
  measures "d97" diameter of A0
  measures "d98" distance of L3.start L3.end
  measures "d99" diameter of A1
extrude "Extrusion17" cut sketch "Sketch18" against normal through all contours A1 A0 | A0 L3 A1 | A2 A0 | A0 A2 | L3 A0 A1
sketch "Sketch19" plane through (50.8, 0, -76.2) normal (1, 0, 0) x (0, 0, -1)
  line L0 (-10.16, 5.08) -> (60.96, 5.08) projected
  line L1 (25.4, 5.08) -> (25.4, 30.48)
  line L2 (50.8, 30.48) -> (0, 30.48) projected
  line L3 (25.4, 17.78) -> (14.1478, 17.78)
  circle A0 centre (14.1478, 17.78) radius 8.89
  circle A1 centre (36.6522, 17.78) radius 8.89
  point P0 (-76.2, 0)
  dimension "d102" = 11.2522
  dimension "d103" = 17.78
  constraints: 4 end point, 3 midpoint, 2 centre point, 1 coincident, 1 horizontal, 1 symmetric about line, 1 other
  measures "d102" distance of L3.start L3.end
  measures "d103" diameter of A0
extrude "Extrusion18" cut sketch "Sketch19" against normal blind 25.4
sketch "Sketch20" plane through (0, 5.08, 0) normal (0, 1, 0) x (1, 0, 0)
  line L0 (50.8, 76.2) -> (38.1, 38.1) projected
  line L1 (50.8, 76.2) -> (49.1936, 71.3807)
  line L2 (49.1936, 71.3807) -> (74.5936, 71.3807)
  line L3 (50.8, 76.2) -> (50.8, 127) projected
  line L4 (50.8, 101.6) -> (58.436, 101.6)
  line L5 (50.8, 127) -> (38.1, 165.1)
  line L6 (49.1936, 131.8193) -> (74.5936, 131.8193)
  line L7 (74.5936, 71.3807) -> (49.1936, 71.3807)
  line L8 (49.1936, 71.3807) -> (49.1936, 131.8193)
  line L9 (49.1936, 131.8193) -> (74.5936, 131.8193)
  line L10 (74.5936, 131.8193) -> (74.5936, 71.3807)
  line L11 (49.1936, 71.3807) -> (38.1, 38.1)
  line L12 (49.1936, 131.8193) -> (38.1, 165.1)
  line L13 (74.5936, 71.3807) -> (69.5136, 71.3807)
  line L14 (69.5136, 71.3807) -> (80.2899, 60.6044)
  line L15 (69.5136, 131.8193) -> (80.2899, 142.5956)
  line L16 (69.5136, 131.8193) -> (84.7536, 131.8193) construction
  line L17 (80.2899, 142.5956) -> (80.2899, 60.6044)
  line L18 (69.5136, 71.3807) -> (61.8936, 71.3807)
  line L19 (61.8936, 71.3807) -> (80.2899, 52.9844)
  line L20 (80.2899, 52.9844) -> (80.2899, 60.6044)
  line L21 (61.8936, 71.3807) -> (61.8936, 131.8193)
  line L22 (69.5136, 131.8193) -> (61.8936, 131.8193)
  line L23 (61.8936, 131.8193) -> (80.2899, 150.2156)
  line L24 (61.8936, 131.8193) -> (87.9099, 131.8193) construction
  line L25 (80.2899, 150.2156) -> (80.2899, 142.5956)
  line L26 (-91.44, 66.04) -> (-91.44, 137.16) projected
  line L27 (-10.16, 137.16) -> (-10.16, 66.04) projected
  line L28 (-91.44, 66.04) -> (-10.16, 66.04)
  line L29 (-10.16, 66.04) -> (-10.16, 137.16)
  line L30 (-10.16, 137.16) -> (-91.44, 137.16)
  line L31 (-91.44, 137.16) -> (-91.44, 66.04)
  line L32 (-10.16, 66.04) -> (-91.44, 66.04)
  line L33 (-91.44, 66.04) -> (-91.44, 137.16)
  line L34 (-91.44, 137.16) -> (-10.16, 137.16)
  line L35 (-10.16, 137.16) -> (-10.16, 66.04)
  line L36 (-10.16, 66.04) -> (-91.44, 137.16) construction
  line L37 (-91.44, 66.04) -> (-10.16, 137.16) construction
  line L38 (-50.8, 203.2) -> (-50.8, 210.836)
  line L39 (-91.7956, 232.6899) -> (-9.8044, 232.6899)
  line L40 (-81.0193, 201.5936) -> (-81.0193, 226.9936)
  line L41 (-81.0193, 226.9936) -> (-20.5807, 226.9936)
  line L42 (-20.5807, 214.2936) -> (-81.0193, 214.2936)
  line L43 (-20.5807, 201.5936) -> (-81.0193, 201.5936)
  line L44 (-25.4, 203.2) -> (-20.5807, 201.5936)
  line L45 (-20.5807, 221.9136) -> (-20.5807, 214.2936)
  line L46 (-20.5807, 201.5936) -> (-20.5807, 226.9936)
  line L47 (-20.5807, 221.9136) -> (-9.8044, 232.6899)
  line L48 (-20.5807, 226.9936) -> (-20.5807, 221.9136)
  line L49 (-2.1844, 232.6899) -> (-9.8044, 232.6899)
  line L50 (-20.5807, 201.5936) -> (12.7, 190.5)
  line L51 (-20.5807, 214.2936) -> (-2.1844, 232.6899)
  line L52 (-20.5807, 226.9936) -> (-20.5807, 201.5936)
  line L53 (-76.2, 203.2) -> (-114.3, 190.5)
  line L54 (-81.0193, 201.5936) -> (-81.0193, 226.9936)
  line L55 (-81.0193, 221.9136) -> (-91.7956, 232.6899)
  line L56 (-81.0193, 221.9136) -> (-81.0193, 214.2936)
  line L57 (-81.0193, 221.9136) -> (-81.0193, 237.1536) construction
  line L58 (-81.0193, 214.2936) -> (-81.0193, 240.3099) construction
  line L59 (-81.0193, 214.2936) -> (-99.4156, 232.6899)
  line L60 (-99.4156, 232.6899) -> (-91.7956, 232.6899)
  line L61 (-81.0193, 201.5936) -> (-114.3, 190.5)
  line L62 (-152.4, 101.6) -> (-160.036, 101.6)
  line L63 (-181.8899, 60.6044) -> (-181.8899, 142.5956)
  line L64 (-150.7936, 71.3807) -> (-176.1936, 71.3807)
  line L65 (-176.1936, 71.3807) -> (-176.1936, 131.8193)
  line L66 (-163.4936, 131.8193) -> (-163.4936, 71.3807)
  line L67 (-150.7936, 131.8193) -> (-150.7936, 71.3807)
  line L68 (-152.4, 127) -> (-150.7936, 131.8193)
  line L69 (-171.1136, 131.8193) -> (-163.4936, 131.8193)
  line L70 (-150.7936, 131.8193) -> (-176.1936, 131.8193)
  line L71 (-171.1136, 131.8193) -> (-181.8899, 142.5956)
  line L72 (-176.1936, 131.8193) -> (-171.1136, 131.8193)
  line L73 (-181.8899, 150.2156) -> (-181.8899, 142.5956)
  line L74 (-150.7936, 131.8193) -> (-139.7, 165.1)
  line L75 (-163.4936, 131.8193) -> (-181.8899, 150.2156)
  line L76 (-176.1936, 131.8193) -> (-150.7936, 131.8193)
  line L77 (-152.4, 76.2) -> (-139.7, 38.1)
  line L78 (-150.7936, 71.3807) -> (-176.1936, 71.3807)
  line L79 (-171.1136, 71.3807) -> (-181.8899, 60.6044)
  line L80 (-171.1136, 71.3807) -> (-163.4936, 71.3807)
  line L81 (-171.1136, 71.3807) -> (-186.3536, 71.3807) construction
  line L82 (-163.4936, 71.3807) -> (-189.5099, 71.3807) construction
  line L83 (-163.4936, 71.3807) -> (-181.8899, 52.9844)
  line L84 (-181.8899, 52.9844) -> (-181.8899, 60.6044)
  line L85 (-150.7936, 71.3807) -> (-139.7, 38.1)
  line L86 (-50.8, 0) -> (-50.8, -7.636)
  line L87 (-9.8044, -29.4899) -> (-91.7956, -29.4899)
  line L88 (-20.5807, 1.6064) -> (-20.5807, -23.7936)
  line L89 (-20.5807, -23.7936) -> (-81.0193, -23.7936)
  line L90 (-81.0193, -11.0936) -> (-20.5807, -11.0936)
  line L91 (-81.0193, 1.6064) -> (-20.5807, 1.6064)
  line L92 (-76.2, 0) -> (-81.0193, 1.6064)
  line L93 (-81.0193, -18.7136) -> (-81.0193, -11.0936)
  line L94 (-81.0193, 1.6064) -> (-81.0193, -23.7936)
  line L95 (-81.0193, -18.7136) -> (-91.7956, -29.4899)
  line L96 (-81.0193, -23.7936) -> (-81.0193, -18.7136)
  line L97 (-99.4156, -29.4899) -> (-91.7956, -29.4899)
  line L98 (-81.0193, 1.6064) -> (-114.3, 12.7)
  line L99 (-81.0193, -11.0936) -> (-99.4156, -29.4899)
  line L100 (-81.0193, -23.7936) -> (-81.0193, 1.6064)
  line L101 (-25.4, 0) -> (12.7, 12.7)
  line L102 (-20.5807, 1.6064) -> (-20.5807, -23.7936)
  line L103 (-20.5807, -18.7136) -> (-9.8044, -29.4899)
  line L104 (-20.5807, -18.7136) -> (-20.5807, -11.0936)
  line L105 (-20.5807, -18.7136) -> (-20.5807, -33.9536) construction
  line L106 (-20.5807, -11.0936) -> (-20.5807, -37.1099) construction
  line L107 (-20.5807, -11.0936) -> (-2.1844, -29.4899)
  line L108 (-2.1844, -29.4899) -> (-9.8044, -29.4899)
  line L109 (-20.5807, 1.6064) -> (12.7, 12.7)
  point P0 (0, 0)
  point P1 (-50.8, 101.6)
  dimension "d106" = 5.08
  dimension "d107" = 25.4
  dimension "d108" = 5.08
  dimension "d109" = 15.24
  dimension "d110" = 45
  dimension "d111" = 45
  dimension "d112" = 7.62
  dimension "d113" = 45
  dimension "d114" = 45
  dimension "d117" = 360
  constraints: 212 end point, 13 point on line, 8 midpoint, 7 horizontal, 6 parallel, 4 collinear, 4 perpendicular, 3 symmetric about line, 2 equal length, 1 vertical, 185 other
  measures "d106" distance of L0.start L1.end
  measures "d107" distance of L1.end L2.end
  measures "d108" distance of L2.end L13.end
  measures "d109" distance of L13.end L14.end
  measures "d110" angle of L14 L13
  measures "d111" angle of L16 L15
  measures "d112" distance of L13.end L18.end
  measures "d113" angle of L19 L18
  measures "d114" angle of L24 L23
extrude "Extrusion19" add sketch "Sketch20" against normal up to surface (5.08 mm away) contours L3 L5 L6 L21 L2 L0 | L21 L6 L10 L2 | L2 L14 L20 L19 | L2 L10 L6 L15 L17 L14 | L23 L25 L15 L6 | L39 L47 L46 L41 L40 L55 | L55 L40 L59 L60 | L49 L51 L45 L47 | L40 L41 L46 L45 L42 | L42 L46 L43 L40 | L63 L71 L70 L65 L64 L79 | L79 L64 L83 L84 | L73 L75 L69 L71 | L64 L65 L70 L69 L66 | L66 L70 L67 L64 | L87 L95 L94 L89 L88 L103 | L103 L88 L107 L108 | L97 L99 L93 L95 | L88 L89 L94 L93 L90 | L90 L94 L91 L88
sketch "Sketch21" plane through (0, 5.08, 0) normal (0, 1, 0) x (1, 0, 0)
  line L0 (-2.1844, -29.4899) -> (-20.5807, -11.0936) projected
  line L1 (61.8936, 71.3807) -> (80.2899, 52.9844) projected
  line L2 (-2.1844, -29.4899) -> (80.2899, 52.9844)
  line L3 (71.0917, 43.7862) -> (73.9982, 59.276)
  point P0 (0, 0)
  constraints: 4 end point, 2 point on line, 1 perpendicular
extrude "Extrusion20" add sketch "Sketch21" along normal blind 25.4
sketch "Sketch22" plane through (80.2899, 5.08, -52.9844) normal (0.7071068, 0, 0.7071068) x (0.7071068, 0, -0.7071068)
  line L0 (-116.6362, 0) -> (-107.6559, 0) projected
  line L1 (-116.6362, 0) -> (-116.6362, 68.58)
  line L2 (0, 0) -> (0, -5.08) projected
  line L3 (0, 0) -> (0, 68.58)
  line L4 (0, 0) -> (68.58, 0) construction
  line L5 (0, 68.58) -> (-116.6362, 68.58)
  arc A0 (-65.0491, 11.43) -> (-51.5871, 11.43) centre (-58.3181, 11.43) ccw projected
  circle A1 centre (-58.3181, 11.43) radius 57.15
  circle A2 centre (-58.3181, 11.43) radius 53.34
  line L6 (-185.3891, 0) -> (-116.6362, 0) projected
  line L7 (-116.6362, 0) -> (-110.4191, 0)
  line L8 (0, 0) -> (-6.2171, 0)
  line L9 (-4.9781, 11.43) -> (-4.9781, 0)
  line L10 (-111.6581, 11.43) -> (-111.6581, 0)
  line L11 (-58.3181, 11.43) -> (-122.9756, 11.43)
  line L12 (-122.9756, 11.43) -> (19.8162, 11.43)
  point P0 (-94.2391, -5.08)
  point P1 (-111.6581, 0)
  point P2 (-2.3228, 0)
  point P3 (-114.3134, 0)
  point P4 (-58.3181, 68.58)
  point P5 (-115.4681, 11.43)
  point P6 (-116.6362, 11.43)
  point P7 (0, 11.43)
  point P8 (-1.1681, 11.43)
  dimension "d123" = 68.58
  dimension "d124" = 68.58
  dimension "d125" = 90
  dimension "d126" = 106.68
  constraints: 20 end point, 5 point on line, 4 point on circle, 3 perpendicular, 3 tangent, 2 centre point, 2 coincident, 2 horizontal, 2 vertical
  measures "d123" distance of L0.start L1.end
  measures "d124" distance of L2.start L3.end
  measures "d125" angle of L4 L3
  measures "d126" diameter of A2
extrude "Extrusion21" add sketch "Sketch22" against normal up to surface (26.0163 mm away) contours L0 A1 L11 L10 | L0 L1 L11 A1 | L11 A1 L12 A2 | L8 L9 L12 A1 | A1 L12 L3 L8
sketch "Sketch25" plane through (80.2899, 5.08, -52.9844) normal (0.7071068, 0, 0.7071068) x (0.7071068, 0, -0.7071068)
  arc A0 (-65.0491, 11.43) -> (-51.5871, 11.43) centre (-58.3181, 11.43) ccw projected
  circle A1 centre (-58.3181, 11.43) radius 54.61
  line L0 (-3.7081, 11.43) -> (-112.9281, 11.43)
  line L1 (-112.9281, 11.43) -> (-112.9281, -30.2508)
  line L2 (-112.9281, -30.2508) -> (-3.7081, -30.2508)
  line L3 (-3.7081, -30.2508) -> (-3.7081, 11.43)
  line L4 (-101.5986, 23.3509) -> (-21.2721, 23.3509)
  line L5 (-21.2721, 23.3509) -> (-21.2721, -25.3148)
  line L6 (-21.2721, -25.3148) -> (-101.5986, -25.3148)
  line L7 (-101.5986, -25.3148) -> (-101.5986, 23.3509)
  circle A2 centre (-58.3181, 11.43) radius 57.15
  line L8 (0, 11.43) -> (0, 25.4) projected
  line L9 (-58.3181, 11.43) -> (0, 11.43)
  line L10 (0, 11.43) -> (0, 25.4)
  line L11 (31.4845, 25.4) -> (-4.4366, 25.4) projected
  line L12 (-2.9018, 25.4) -> (0, 25.4)
  point P0 (-94.2391, -5.08)
  point P1 (-112.9281, 11.43)
  point P2 (-98.717, -25.3148)
  point P3 (-101.5986, -21.8725)
  point P4 (-1.1681, 11.43)
  dimension "d134" = 109.22
  constraints: 22 end point, 4 parallel, 3 horizontal, 3 perpendicular, 2 coincident, 2 point on line, 1 collinear, 6 other
extrude "Extrusion24" cut sketch "Sketch25" against normal up to surface (26.0163 mm away) contours L7 A1 L0 | L0 A1 L5 L4 L7 | L0 A1 L2 L6 L5 | A1 L7 L6 L2 A2 L1 | A1 L6 L7 | L3 A2 L2 A1 | A2 L2 L1 | L3 L2 A2 | A2 L11 L8 L9
sketch "Sketch26" plane through (-20.5807, 5.08, 11.0936) normal (0, -1, 0) x (0.7071068, 0, -0.7071068)
  line L0 (3.7081, 0) -> (3.7081, 26.0163) projected
  line L1 (3.7081, 26.0163) -> (0, 26.0163)
  line L2 (0, 26.0163) -> (0, -5.415)
  line L3 (0, -5.415) -> (3.7081, -5.415)
  line L4 (3.7081, -5.415) -> (3.7081, 26.0163)
  line L5 (112.9281, 26.0163) -> (112.9281, 0) projected
  line L6 (112.9281, 26.0163) -> (116.6362, 26.0163)
  line L7 (116.6362, 26.0163) -> (116.6362, -7.7655)
  line L8 (116.6362, -7.7655) -> (112.9281, -7.7655)
  line L9 (112.9281, -7.7655) -> (112.9281, 26.0163)
  point P0 (22.3971, 6.7084)
  point P1 (3.7081, 0)
  constraints: 16 end point, 4 parallel, 2 horizontal, 2 perpendicular
extrude "Extrusion25" add sketch "Sketch26" along normal up to surface (5.08 mm away)
sketch "Sketch27" plane through (80.2899, 0, -52.9844) normal (0.7071068, 0, 0.7071068) x (0.7071068, 0, -0.7071068)
  arc A0 (-65.0491, 16.51) -> (-51.5871, 16.51) centre (-58.3181, 16.51) ccw projected
  circle A1 centre (-58.3181, 16.51) radius 57.15
  line L0 (-116.6362, 5.08) -> (-116.6362, 16.51) projected
  circle A2 centre (-58.3181, 16.51) radius 58.3181
  line L1 (0, 16.51) -> (0, 5.08) projected
  line L2 (-116.6362, 16.51) -> (0, 16.51)
  point P0 (-94.2391, 0)
  point P1 (-1.1681, 16.51)
  point P2 (-115.4681, 16.51)
  constraints: 2 centre point, 2 coincident, 2 end point, 1 horizontal, 1 point on circle
extrude "Extrusion26" add sketch "Sketch27" against normal up to surface (26.0163 mm away) contours L2 A2 A1 picked at (-90.178, 64.6266)
sketch "Sketch28" plane through (0, 5.08, 0) normal (0, 1, 0) x (1, 0, 0)
  line L0 (-2.1844, -29.4899) -> (-20.5807, -11.0936) projected
  line L1 (-17.9587, -8.4715) -> (-20.5807, -11.0936) projected
  line L2 (-2.1844, -29.4899) -> (-20.5807, -11.0936)
  line L3 (-20.5807, -11.0936) -> (61.8936, 71.3807)
  line L4 (61.8936, 71.3807) -> (80.2899, 52.9844)
  line L5 (80.2899, 52.9844) -> (-2.1844, -29.4899)
  line L6 (12.7, 12.7) -> (38.1, 38.1) projected
  line L7 (12.7, 12.7) -> (-15.8371, -15.8371)
  line L8 (-15.8371, -15.8371) -> (66.6371, 66.6371)
  line L9 (-91.44, 137.16) -> (-91.44, 66.04) projected
  line L10 (-10.16, 66.04) -> (-10.16, 137.16) projected
  line L11 (-91.44, 66.04) -> (-10.16, 66.04)
  line L12 (-10.16, 66.04) -> (-10.16, 137.16)
  line L13 (-10.16, 137.16) -> (-91.44, 137.16)
  line L14 (-91.44, 137.16) -> (-91.44, 66.04)
  circle A0 centre (-50.8, 101.6) radius 54.0011
  line L15 (80.2899, 150.2156) -> (61.8936, 131.8193)
  line L16 (61.8936, 131.8193) -> (-20.5807, 214.2936)
  line L17 (-20.5807, 214.2936) -> (-2.1844, 232.6899)
  line L18 (66.6371, 136.5629) -> (-15.8371, 219.0371)
  line L19 (-2.1844, 232.6899) -> (80.2899, 150.2156)
  line L20 (38.1, 165.1) -> (66.6371, 136.5629)
  line L21 (-99.4156, 232.6899) -> (-81.0193, 214.2936)
  line L22 (-81.0193, 214.2936) -> (-163.4936, 131.8193)
  line L23 (-163.4936, 131.8193) -> (-181.8899, 150.2156)
  line L24 (-85.7629, 219.0371) -> (-168.2371, 136.5629)
  line L25 (-181.8899, 150.2156) -> (-99.4156, 232.6899)
  line L26 (-114.3, 190.5) -> (-85.7629, 219.0371)
  line L27 (-181.8899, 52.9844) -> (-163.4936, 71.3807)
  line L28 (-163.4936, 71.3807) -> (-81.0193, -11.0936)
  line L29 (-81.0193, -11.0936) -> (-99.4156, -29.4899)
  line L30 (-168.2371, 66.6371) -> (-85.7629, -15.8371)
  line L31 (-99.4156, -29.4899) -> (-181.8899, 52.9844)
  line L32 (-139.7, 38.1) -> (-168.2371, 66.6371)
  point P0 (0, 0)
  point P1 (-15.24, 142.24)
  point P2 (-91.44, 137.16)
  point P3 (-86.36, 60.96)
  dimension "d143" = 360
  constraints: 56 end point, 12 point on line, 4 parallel, 4 perpendicular, 1 horizontal, 60 other
extrude "Extrusion27" add sketch "Sketch28" along normal blind 69.7484 contours L15 L18 L17 L19 | L21 L24 L23 L25 | L27 L30 L29 L31
sketch "Sketch30" plane through (-2.1844, 5.08, -232.6899) normal (0.7071068, 0, -0.7071068) x (-0.7071068, 0, -0.7071068)
  line L0 (-163.5412, 11.43) -> (-151.0952, 11.43) projected
  line L1 (-163.5412, 11.43) -> (18.5829, 11.43)
  line L2 (-116.6362, 0) -> (-116.6362, -5.08) projected
  line L3 (-116.6362, 0) -> (-112.9278, 0)
  line L4 (-112.9278, 0) -> (-112.9278, 11.43)
  line L5 (-112.9278, 11.43) -> (-116.6362, 11.43)
  line L6 (-116.6362, 11.43) -> (-116.6362, 0)
  arc A0 (-65.0491, 11.43) -> (-51.5871, 11.43) centre (-58.3181, 11.43) ccw projected
  circle A1 centre (-58.3181, 11.43) radius 54.6097
  circle A2 centre (-58.3181, 11.43) radius 58.3181
  line L7 (0, 0) -> (0, 69.7484) projected
  line L8 (-116.6362, 0) -> (0, 0)
  line L9 (0, 0) -> (0, 69.7484)
  line L10 (0, 69.7484) -> (-116.6362, 69.7484)
  line L11 (-116.6362, 69.7484) -> (-116.6362, 0)
  line L12 (0, 0) -> (-8.9803, 0) projected
  line L13 (0, 0) -> (-3.7084, 0)
  line L14 (-3.7084, 0) -> (-3.7084, 11.43)
  line L15 (-3.7084, 11.43) -> (0, 11.43)
  line L16 (0, 11.43) -> (0, 0)
  point P0 (-166.0812, -5.08)
  point P1 (-3.7084, 0)
  point P2 (-112.9278, 0)
  point P3 (-116.6362, 11.43)
  point P4 (0, 11.43)
  dimension "d147" = 3.7084
  constraints: 26 end point, 6 parallel, 3 horizontal, 3 perpendicular, 2 coincident, 2 point on circle, 2 point on line, 1 centre point, 1 collinear, 3 other
  measures "d147" distance of L5.end L4.end
extrude "Extrusion28" cut sketch "Sketch30" against normal up to surface (19.3079 mm away) contours L11 L10 A2 | A1 L1 | A1 L8 L4 | L1 A0 A1 L8 | L10 L7 A2 | L1 A0 | L14 L8 A1
sketch "Sketch31" plane through (-181.8899, 5.08, -150.2156) normal (-0.7071068, 0, -0.7071068) x (-0.7071068, 0, 0.7071068)
  arc A0 (-65.0491, 11.43) -> (-51.5871, 11.43) centre (-58.3181, 11.43) ccw projected
  circle A1 centre (-58.3181, 11.43) radius 54.61
  circle A2 centre (-58.3181, 11.43) radius 58.3181
  line L0 (-116.6362, 0) -> (-116.6362, 69.7484) projected
  line L1 (-185.3891, 0) -> (-116.6362, 0) projected
  line L2 (-116.6362, 0) -> (-112.9281, 0)
  line L3 (-112.9281, 0) -> (-112.9281, 11.43)
  line L4 (-112.9281, 11.43) -> (-116.6362, 11.43)
  line L5 (-116.6362, 11.43) -> (-116.6362, 0)
  line L6 (0, 0) -> (-3.7081, 0)
  line L7 (-3.7081, 0) -> (-3.7081, 11.43)
  line L8 (-3.7081, 11.43) -> (0, 11.43)
  line L9 (0, 11.43) -> (0, 0)
  line L10 (0, 11.43) -> (-116.6362, 11.43)
  line L11 (-116.6362, 69.7484) -> (0, 69.7484) projected
  line L12 (-116.6362, 0) -> (0, 0)
  line L13 (0, 0) -> (0, 69.7484)
  line L14 (0, 69.7484) -> (-116.6362, 69.7484)
  line L15 (-116.6362, 69.7484) -> (-116.6362, 0)
  point P0 (-22.3971, -5.08)
  point P1 (-3.7081, 0)
  point P2 (-112.9281, 0)
  point P3 (0, 11.43)
  point P4 (-116.6362, 11.43)
  dimension "d150" = 109.22
  constraints: 26 end point, 6 parallel, 3 horizontal, 3 perpendicular, 2 centre point, 2 coincident, 2 point on circle, 2 point on line, 1 collinear, 1 tangent
  measures "d150" diameter of A1
extrude "Extrusion29" cut sketch "Sketch31" against normal up to surface (19.3079 mm away) contours L10 A0 | L10 A1 | A0 L10 A1 L12 | A1 L12 L3 | L7 L12 A1 | L0 L11 A2 | A2 L11 L13